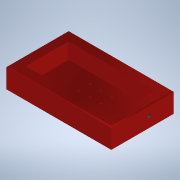
# Autodesk Inventor part: UNLHEP-14-01-P-004_ChuckForGantry
Saved by Autodesk Inventor 2022 (Build 260153000, 153)
## iProperties
Created: 2014-01-09
Part Number: UNLHEP-14-01-P-004_ChuckForGantry
Material: Aluminum, Anodized Red
Document SubType Name: Modeling
Designer: Frank Meier
Density: 2.7 g/cm^3
Project: UNL Pixel Phase I
Mass: 2699.72 g
Surface Area: 1115.91 cm^2
Volume: 999.896 cm^3
Appearance: Anodized - Red
Author: Frank Meier
Revision Number: 00
Autodesk Inventor part; units mm, degrees
ref_plane "YZ Plane" through (0, 0, 0) normal (1, 0, 0) x (0, 1, 0)
ref_plane "XZ Plane" through (0, 0, 0) normal (0, 1, 0) x (-1, 0, 0)
ref_plane "XY Plane" through (0, 0, 0) normal (0, 0, 1) x (1, 0, 0)
sketch "Skizze1" plane through (0, 0, 0) normal (0, 0, 1) x (1, 0, 0)
  line L0 (-117.475, -69.85) -> (117.475, -69.85)
  line L1 (117.475, -69.85) -> (117.475, 69.85)
  line L2 (117.475, 69.85) -> (-117.475, 69.85)
  line L3 (-117.475, 69.85) -> (-117.475, -69.85)
  line L4 (-117.475, -69.85) -> (117.475, 69.85) construction
  line L5 (117.475, -69.85) -> (-117.475, 69.85) construction
  point P0 (0, 0)
  dimension "d0" = 234.95
  dimension "d2" = 139.7
  constraints: 12 end point, 2 midpoint, 2 parallel, 1 horizontal, 1 perpendicular
  measures "d0" distance of L1.end L2.end
  measures "d2" distance of L0.end L1.end
extrude "Extrusion1" add sketch "Skizze1" along normal blind 44.45
sketch "Skizze2" plane through (0, 0, 44.45) normal (0, 0, 1) x (1, 0, 0)
  line L0 (-96, -48) -> (96, -48)
  line L1 (96, -48) -> (96, 48)
  line L2 (96, 48) -> (-96, 48)
  line L3 (-96, 48) -> (-96, -48)
  line L4 (-96, -48) -> (96, 48) construction
  line L5 (96, -48) -> (-96, 48) construction
  point P0 (0, 0)
  dimension "d5" = 192
  dimension "d7" = 96
  constraints: 12 end point, 2 midpoint, 2 parallel, 1 horizontal, 1 perpendicular
  measures "d5" distance of L1.end L2.end
  measures "d7" distance of L0.end L1.end
extrude "Extrusion2" cut sketch "Skizze2" against normal blind 36
fillet "Rundung1" radius 4 4 edges at (-96, 48, 26.45) (96, 48, 26.45) (96, -48, 26.45) (-96, -48, 26.45)
chamfer "Fase1" distance 2 angle 45 4 edges at (0, -69.85, 44.45) (-117.475, 0, 44.45) (0, 69.85, 44.45) (117.475, 0, 44.45)
sketch "Skizze4" plane through (0, 0, 44.45) normal (0, 0, 1) x (1, 0, 0)
  line L0 (117.475, 69.85) -> (-117.475, 69.85) projected
  line L1 (117.475, -69.85) -> (117.475, 69.85) projected
  line L2 (-117.475, 69.85) -> (-117.475, -69.85) projected
  line L3 (-117.475, -69.85) -> (117.475, -69.85) projected
  point P0 (-112.475, 45.85)
  point P1 (-112.475, -45.85)
  point P2 (-93.475, -64.85)
  point P3 (-93.475, 64.85)
  point P4 (93.475, 64.85)
  point P5 (112.475, 45.85)
  point P6 (112.475, -45.85)
  point P7 (93.475, -64.85)
  dimension "d153" = 24
  dimension "d154" = 24
  dimension "d155" = 5
  dimension "d156" = 5
  dimension "d157" = 24
  dimension "d158" = 5
  dimension "d159" = 5
  dimension "d160" = 24
  dimension "d161" = 24
  dimension "d162" = 5
  dimension "d163" = 5
  dimension "d164" = 24
  dimension "d165" = 5
  dimension "d166" = 24
  dimension "d167" = 5
  dimension "d168" = 24
  measures "d153" distance from line of L0 point (-112.475, 45.85)
  measures "d154" distance from line of L3 point (-112.475, -45.85)
  measures "d155" distance from line of L2 point (-112.475, -45.85)
  measures "d156" distance from line of L3 point (-93.475, -64.85)
  measures "d157" distance from line of L2 point (-93.475, -64.85)
  measures "d158" distance from line of L2 point (-112.475, 45.85)
  measures "d159" distance from line of L0 point (-93.475, 64.85)
  measures "d160" distance from line of L2 point (-93.475, 64.85)
  measures "d161" distance from line of L1 point (93.475, 64.85)
  measures "d162" distance from line of L0 point (93.475, 64.85)
  measures "d163" distance from line of L1 point (112.475, 45.85)
  measures "d164" distance from line of L0 point (112.475, 45.85)
  measures "d165" distance from line of L1 point (112.475, -45.85)
  measures "d166" distance from line of L3 point (112.475, -45.85)
  measures "d167" distance from line of L3 point (93.475, -64.85)
  measures "d168" distance from line of L1 point (93.475, -64.85)
hole "Bohrung7" at (-112.475, 45.85, 44.45) at (-112.475, -45.85, 44.45) at (-93.475, -64.85, 44.45) at (-93.475, 64.85, 44.45) at (93.475, 64.85, 44.45) at (112.475, 45.85, 44.45) at (112.475, -45.85, 44.45) at (93.475, -64.85, 44.45) direction (0, 0, -1) diameter 3.242 depth 20 tip angle 118 thread size "M4x0.7" class "6H" standard "ISO Metric profile"
sketch "Sketch12" plane through (0, 0, 8.45) normal (0, 0, 1) x (1, 0, 0)
  line L0 (-115.475, 67.85) -> (115.475, 67.85) projected
  line L1 (-115.475, -67.85) -> (-115.475, 67.85) projected
  point P0 (0, 0)
  point P1 (-25, 25)
  point P2 (0, 25)
  point P3 (25, 25)
  point P4 (-25, 0)
  point P5 (0, 0)
  point P6 (25, 0)
  point P7 (-25, -25)
  point P8 (0, -25)
  point P9 (25, -25)
  dimension "d217" = 25
  dimension "d218" = 25
  dimension "d221" = 25
  dimension "d224" = 25
  constraints: 1 horizontal, 1 vertical, 8 other
  measures "d217" horizontal distance of point (0, 0) point (-25, 25)
  measures "d218" horizontal distance of point (0, 0) point (-25, 25)
  measures "d221" distance of point (-25, 25) point (0, 25)
  measures "d224" distance of point (-25, 25) point (-25, 0)
sketch "Sketch13" plane through (117.475, -69.85, 0) normal (1, 0, 0) x (0, 0, -1)
  line L0 (0, 139.7) -> (-42.45, 139.7) projected
  line L1 (0, 0) -> (0, 139.7) projected
  point P0 (0, 69.85)
  point P1 (-23, 84.7)
  dimension "d206" = 55
  dimension "d207" = 23
  measures "d206" distance from line of L0 point (-23, 84.7)
  measures "d207" distance from line of L1 point (-23, 84.7)
hole "Hole10" at (117.475, 14.85, 23) direction (-1, 0, 0) diameter 7.95 depth 21.475 tip angle 118 taper from width 8.7366 to width 8.304 over 6.924 thread size "1/8" designation "1/8 - 27 NPT" standard "NPT"
hole "Hole11" at (-25, 25, 8.45) at (0, 25, 8.45) at (25, 25, 8.45) at (-25, 0, 8.45) at (0, 0, 8.45) at (25, 0, 8.45) at (-25, -25, 8.45) at (0, -25, 8.45) at (25, -25, 8.45) direction (0, 0, -1) diameter 5.105 end through all clearance for "Flat Head Machine Screw (82)" size "#10" standard "Ansi Unified Screw Threads"
